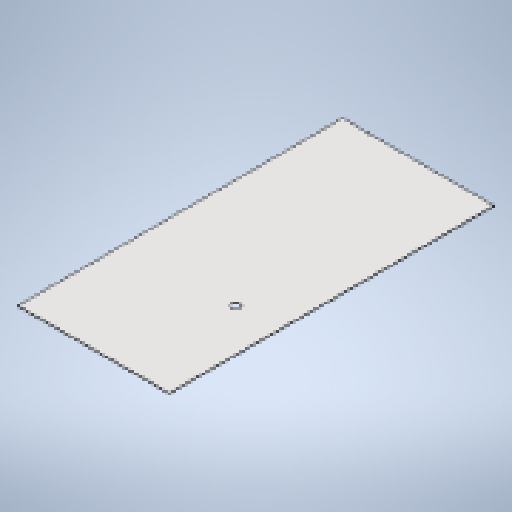
# Autodesk Inventor part: GnG frame 2 floor sheet 10
Saved by Autodesk Inventor 2025 (Build 290162010, 162A)
## iProperties
Created: 2025-10-28
Part Number: GnG frame 2 floor sheet 10
Material: Stainless Steel
Document SubType Name: Sheet Metal
Designer: admin
Mass: 280.619 g
Surface Area: 364.406 cm^2
Volume: 35.0774 cm^3
Density: 8 g/cm^3
Sheet Metal Rule: AISI304 3mm Die 32
Sheet Metal Width: 700,000 mm
Sheet Metal Length: 1500,000 mm
Sheet Metal Area: 1050000,000 mm^2
Appearance: Default
Flat Pattern Width: 70 cm
Flat Pattern Length: 150 cm
Flat Pattern Area: 10500 cm^2
Author: admin
Autodesk Inventor part; units mm, degrees
ref_plane "YZ Plane" through (0, 0, 0) normal (1, 0, 0) x (0, 1, 0)
ref_plane "XZ Plane" through (0, 0, 0) normal (0, 1, 0) x (-1, 0, 0)
ref_plane "XY Plane" through (0, 0, 0) normal (0, 0, 1) x (1, 0, 0)
sketch "Sketch1" plane through (0, 0, 0) normal (0, 0, 1) x (1, 0, 0)
  line L0 (0, 0) -> (-700, 0)
  line L1 (-700, 0) -> (-700, -1500)
  line L2 (-700, -1500) -> (0, -1500)
  line L3 (0, -1500) -> (0, 0)
  line L4 (0, 0) -> (-40, 0)
  line L5 (-40, 0) -> (-40, -35)
  line L6 (-40, -35) -> (0, -35)
  line L7 (0, -35) -> (0, 0)
  line L8 (0, -1500) -> (-40, -1500)
  line L9 (-40, -1500) -> (-40, -1465)
  line L10 (-40, -1465) -> (0, -1465)
  line L11 (0, -1465) -> (0, -1500)
  line L12 (-700, 0) -> (-660, 0)
  line L13 (-660, 0) -> (-660, -35)
  line L14 (-660, -35) -> (-700, -35)
  line L15 (-700, -35) -> (-700, 0)
  line L16 (-700, -1500) -> (-660, -1500)
  line L17 (-660, -1500) -> (-660, -1465)
  line L18 (-660, -1465) -> (-700, -1465)
  line L19 (-700, -1465) -> (-700, -1500)
  line L20 (-240, -1500) -> (-140, -1500)
  line L21 (-140, -1500) -> (-140, -1465)
  line L22 (-140, -1465) -> (-240, -1465)
  line L23 (-240, -1465) -> (-240, -1500)
  line L24 (-240, 0) -> (-140, 0)
  line L25 (-140, 0) -> (-140, -35)
  line L26 (-140, -35) -> (-240, -35)
  line L27 (-240, -35) -> (-240, 0)
  point P0 (0, -35)
  point P1 (-40, 0)
  point P2 (0, -1465)
  point P3 (-140, 0)
  point P4 (-660, 0)
  point P5 (-700, -35)
  point P6 (-700, -1465)
  point P7 (-660, -1500)
  point P8 (-300, -35)
  point P9 (-300, 0)
  point P10 (-260, -2265)
  point P11 (-260, -2300)
  point P12 (-260, -35)
  point P13 (-260, 0)
  point P14 (-300, -2265)
  point P15 (-300, -2300)
  point P16 (-240, 0)
  dimension "d22" = 700
  dimension "d23" = 1500
  dimension "d24" = 40
  dimension "d25" = 35
  dimension "d28" = 100
  dimension "d29" = 100
  measures "d22" distance of L2.end L1.end
  measures "d23" distance of L1.end L0.end
  measures "d24" distance of L6.end L5.end
  measures "d25" distance of L5.end L4.end
  measures "d28" distance of L25.end L26.end
  measures "d29" distance between parallel lines of L5 L25
extrude "Plate1" add sketch "Sketch1" along normal blind 3
sketch "Sketch5" plane through (0, 0, 0) normal (0, 0, -1) x (-1, 0, 0)
  line L0 (700, 0) -> (600, 0) construction
  line L1 (600, 0) -> (600, -2) construction
  line L2 (600, -2) -> (700, -2) construction
  line L3 (700, -2) -> (700, 0) construction
  line L4 (600, 0) -> (598.4752, -4.6556)
  arc A0 (597.5248, -4.6556) -> (598.4752, -4.6556) centre (598, -4.5) ccw
  line L5 (597.5248, -4.6556) -> (596, 0)
  line L6 (596, 0) -> (600, 0)
  line L7 (596, 0) -> (594, 0) construction
  line L8 (594, 0) -> (592, 0)
  line L9 (592, 0) -> (592, -5)
  line L10 (592, -5) -> (594, -5)
  line L11 (594, -5) -> (594, 0)
  line L12 (592, 0) -> (590, 0) construction
  line L13 (590, 0) -> (588, 0)
  line L14 (588, 0) -> (588, -5)
  line L15 (588, -5) -> (590, -5)
  line L16 (590, -5) -> (590, 0)
  line L17 (588, 0) -> (586, 0) construction
  line L18 (586, 0) -> (584, 0)
  line L19 (584, 0) -> (584, -5)
  line L20 (584, -5) -> (586, -5)
  line L21 (586, -5) -> (586, 0)
  line L22 (584, 0) -> (582, 0) construction
  line L23 (582, 0) -> (580, 0)
  line L24 (580, 0) -> (580, -5)
  line L25 (580, -5) -> (582, -5)
  line L26 (582, -5) -> (582, 0)
  line L27 (580, 0) -> (575, 0) construction
  line L28 (575, 0) -> (570, 0) construction
  circle A1 centre (575, 0) radius 1
  circle A2 centre (570, 0) radius 1
  point P0 (0, 0)
  point P1 (598, 0)
  dimension "d30" = 100
  dimension "d31" = 2
  dimension "d32" = 5
  dimension "d33" = 4
  dimension "d34" = 0.5
  dimension "d35" = 5
  dimension "d36" = 5
  dimension "d37" = 5
  dimension "d38" = 2
  constraints: 58 end point, 11 horizontal, 10 equal length, 10 parallel, 5 perpendicular, 4 coincident, 3 centre point, 3 tangent, 2 point on circle, 1 equal radius, 1 midpoint, 1 point on line, 1 vertical alignment
  measures "d30" distance of L2.end L1.end
  measures "d31" distance of L1.end L0.end
  measures "d32" distance of L9.end L9.start
  measures "d33" distance of L5.end L0.end
  measures "d34" radius of A0
  measures "d35" distance of L15.start L13.end
  measures "d36" distance of L19.end L19.start
  measures "d37" distance of L24.end L24.start
  measures "d38" diameter of A1
extrude "Cut1" cut sketch "Sketch5" against normal blind 3 contours L26 L25 L24 L23 | A1 | A2
sketch "Sketch6" plane through (0, 0, 0) normal (0, 0, -1) x (-1, 0, 0)
  circle A0 centre (194.6369, -998.5751) radius 19.7563
  point P0 (0, 0)
  constraints: 1 centre point
extrude "Cut2" cut sketch "Sketch6" against normal blind 3
equation "\"d33\" = 2 * d31"
equation "\"d34\" = 0.25 * d31"
equation "\"d38\" = d31"
equation "\"d39\" = Thickness"
equation "\"d41\" = Thickness"
equation "\"d2\" = Thickness"
equation "\"BendReliefWidth\" = Thickness"
equation "\"BendReliefDepth\" = 0.5 * Thickness"
equation "\"CornerReliefSize\" = 4 * Thickness"
equation "\"MinimumRemnant\" = 2 * Thickness"
equation "\"TransitionRadius\" = BendRadius"
equation "\"JacobiRadiusSize\" = BendRadius"
equation "\"GapSize\" = Thickness"
equation "\"Thickness\" = 3"
equation "\"BendRadius\" = 5"
body "Solid1"
